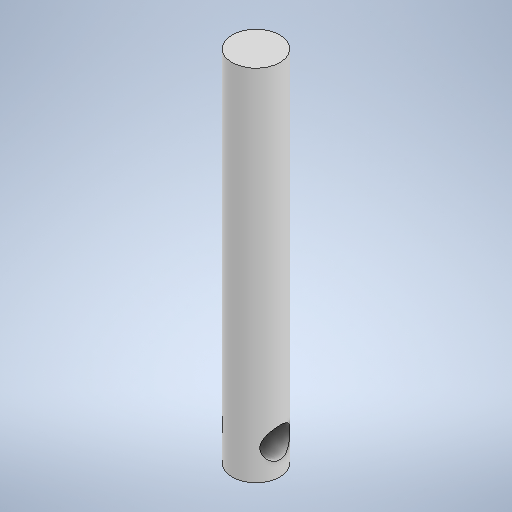
# Autodesk Inventor part: rod2
Saved by Autodesk Inventor 2025.2 (Build 292293000, 293)
## iProperties
Created: 2026-01-09
Part Number: rod2
Material: Generic
Document SubType Name: Modeling
Designer: William
Density: 1 g/cm^3
Appearance: Default
Author: William
Autodesk Inventor part; units mm, degrees
ref_plane "XZ Plane" through (0, 0, 0) normal (0, 1, 0) x (-1, 0, 0)
ref_plane "XY Plane" through (0, 0, 0) normal (0, 0, 1) x (1, 0, 0)
sketch "Sketch1" plane through (0, 0, 0) normal (0, 1, 0) x (-1, 0, 0)
  circle A0 centre (0, 0) radius 4
  dimension "d0" = 8
  constraints: 1 centre point, 1 coincident
  measures "d0" diameter of A0
extrude "Extrusion1" add sketch "Sketch1" along normal blind 60
sketch "Sketch2" plane through (0, 0, 0) normal (1, 0, 0) x (0, 1, 0)
  circle A0 centre (5, 0) radius 2.5
  line L0 (0, -4) -> (0, 4) projected
  point P0 (0, 0)
  dimension "d3" = 5
  dimension "d4" = 5
  constraints: 1 centre point
  measures "d3" diameter of A0
  measures "d4" distance from line of L0 A0.centre
extrude "Extrusion2" cut sketch "Sketch2" along normal mid plane 50
ref_plane "Work Plane1" through (-4, 0, 0) normal (1, 0, 0) x (0, 1, 0)
body "Solid1"
